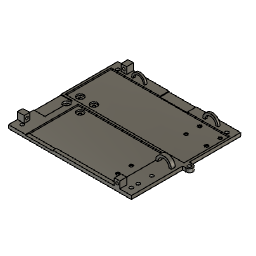
cocheV3 v2 (Autodesk Fusion 360 design; units mm, degrees)
Autodesk Fusion 360 part; units mm, degrees
sketch "Sketch1" plane through (0, 0, 0) normal (0, 0, 1) x (1, 0, 0)
  line L0 (-100, 120) -> (80, 120)
  line L1 (80, 120) -> (80, -40)
  line L2 (80, -40) -> (-100, -40)
  line L3 (-100, -40) -> (-100, 120)
  line L4 (80, 120) -> (80, 110)
  circle A0 centre (70, 110) radius 2
  circle A1 centre (70, -30) radius 2
  circle A2 centre (-90, 110) radius 2
  circle A3 centre (-90, -30) radius 2
  dimension "d1" = 180
  dimension "d2" = 160
  dimension "d3" = 4
  dimension "d4" = 4
  dimension "d5" = 4
  dimension "d6" = 4
  constraint horizontal L0
  constraint vertical L1
  constraint horizontal L2
  constraint vertical L3
  constraint coincident L1 L4.end
  measures "d1" distance of L0.start L0.end
  measures "d2" distance of L0.start L2.end
  measures "d3" diameter of A0
  measures "d4" diameter of A1
  measures "d5" diameter of A2
  measures "d6" diameter of A3
extrude "Extrude1" add sketch "Sketch1" along normal blind 5 contours L0 L1 L2 L3 L4 | A0 | A1 | A2 | A3
sketch "Sketch2" plane through (0, 0, 5) normal (0, 0, 1) x (-1, 0, 0)
  line L0 (-80, -120) -> (100, -120)
  line L1 (100, -120) -> (100, 40)
  line L2 (100, 40) -> (-80, 40)
  line L3 (-80, 40) -> (-80, -120)
  circle A0 centre (-70, -110) radius 2
  circle A1 centre (-70, 30) radius 2
  circle A2 centre (90, -110) radius 2
  circle A3 centre (90, 30) radius 2
  dimension "d9" = 4
  dimension "d10" = 4
  dimension "d11" = 4
  dimension "d12" = 4
  measures "d9" diameter of A0
  measures "d10" diameter of A1
  measures "d11" diameter of A2
  measures "d12" diameter of A3
extrude "Extrude2" add sketch "Sketch2" along normal blind 40 contours A0 | A1 | A2 | A3
sketch "Sketch3" plane through (0, 0, 5) normal (0, 0, 1) x (-1, 0, 0)
  circle A0 centre (90, 30) radius 2
  circle A1 centre (-70, 30) radius 2
  circle A2 centre (90, -110) radius 2
  circle A3 centre (-70, -110) radius 2
  line L0 (-80, -120) -> (100, -120)
  line L1 (100, -120) -> (100, 40)
  line L2 (100, 40) -> (-80, 40)
  line L3 (-80, 40) -> (-80, -120)
  line L4 (-77, -107) -> (97, -107)
  line L5 (97, -107) -> (97, -40)
  line L6 (97, -40) -> (-77, -40)
  line L7 (-77, -40) -> (-77, -107)
  line L8 (75, 35) -> (-53, 35)
  line L9 (-53, 35) -> (-53, -37)
  line L10 (-53, -37) -> (75, -37)
  line L11 (75, -37) -> (75, 35)
  dimension "d15" = 67
  dimension "d16" = 174
  dimension "d17" = 128
  dimension "d18" = 72
  constraint horizontal L4
  constraint vertical L5
  constraint horizontal L6
  constraint vertical L7
  constraint horizontal L8
  constraint vertical L9
  constraint horizontal L10
  constraint vertical L11
  measures "d15" distance of L4.start L6.end
  measures "d16" distance of L4.start L4.end
  measures "d17" distance of L8.start L8.end
  measures "d18" distance of L8.start L10.end
extrude "Extrude3" cut sketch "Sketch3" against normal blind 2 contours L4 L5 L6 L7 | L8 L9 L10 L11
sketch "Sketch4" plane through (0, 0, 5) normal (0, 0, 1) x (-1, 0, 0)
  line L0 (97, -107) -> (-77, -107)
  line L1 (-77, -107) -> (-77, -40)
  line L2 (-77, -40) -> (97, -40)
  line L3 (97, -40) -> (97, -107)
  line L4 (-53, 35) -> (75, 35)
  line L5 (75, 35) -> (75, -37)
  line L6 (75, -37) -> (-53, -37)
  line L7 (-53, -37) -> (-53, 35)
  circle A0 centre (90, 30) radius 2
  circle A1 centre (-70, 30) radius 2
  circle A2 centre (90, -110) radius 2
  circle A3 centre (-70, -110) radius 2
  line L8 (-80, -120) -> (100, -120)
  line L9 (100, -120) -> (100, 40)
  line L10 (100, 40) -> (-80, 40)
  line L11 (-80, 40) -> (-80, -120)
  line L12 (-80, -120) -> (-80, -70)
  line L13 (-80, -70) -> (-77, -70)
  circle A4 centre (-70, -80) radius 1.5
  circle A5 centre (-40, -80) radius 1.5
  circle A6 centre (-70, -100) radius 1.5
  circle A7 centre (-40, -100) radius 1.5
  circle A8 centre (-40, 20) radius 1.5
  circle A9 centre (-40, 0) radius 1.5
  circle A10 centre (-70, 20) radius 1.5
  circle A11 centre (-70, 0) radius 1.5
  point P0 (-40, 0)
  point P1 (-40, 20)
  point P2 (-70, 0)
  point P3 (-70, 20)
  dimension "d21" = 50
  dimension "d23" = 3
  dimension "d24" = 3
  dimension "d25" = 3
  dimension "d26" = 3
  dimension "d27" = 3
  dimension "d28" = 3
  dimension "d29" = 3
  dimension "d30" = 3
  constraint coincident L8.start L11.end
  constraint coincident L11 L12.end
  constraint perpendicular L1 L13
  constraint coincident L1 L13.end
  constraint symmetric L2 A4.centre P2
  constraint symmetric L2 A5.centre P0
  constraint symmetric L2 A6.centre P3
  constraint symmetric L2 A7.centre P1
  constraint coincident P1 A8.centre
  constraint coincident P0 A9.centre
  constraint coincident P3 A10.centre
  constraint coincident P2 A11.centre
  measures "d21" distance of L8.start L12.end
  measures "d23" diameter of A4
  measures "d24" diameter of A5
  measures "d25" diameter of A6
  measures "d26" diameter of A7
  measures "d27" diameter of A8
  measures "d28" diameter of A9
  measures "d29" diameter of A10
  measures "d30" diameter of A11
extrude "Extrude4" cut sketch "Sketch4" against normal blind 5 contours A4 | A5 | A6 | A7 | A8 | A9 | A10 | A11
sketch "Sketch5" plane through (0, 0, 5) normal (0, 0, 1) x (-1, 0, 0)
  circle A0 centre (-70, 20) radius 1.5
  circle A1 centre (-70, 0) radius 1.5
  line L0 (97, -107) -> (-77, -107)
  line L1 (-77, -107) -> (-77, -40)
  line L2 (-77, -40) -> (97, -40)
  line L3 (97, -40) -> (97, -107)
  line L4 (-53, 35) -> (75, 35)
  line L5 (75, 35) -> (75, -37)
  line L6 (75, -37) -> (-53, -37)
  line L7 (-53, -37) -> (-53, 35)
  circle A2 centre (90, 30) radius 2
  circle A3 centre (-70, 30) radius 2
  circle A4 centre (90, -110) radius 2
  circle A5 centre (-70, -110) radius 2
  line L8 (-80, -120) -> (100, -120)
  line L9 (100, -120) -> (100, 40)
  line L10 (100, 40) -> (-80, 40)
  line L11 (-80, 40) -> (-80, -120)
  circle A6 centre (-40, -100) radius 2.5
  circle A7 centre (-70, -100) radius 2.5
  circle A8 centre (-40, -80) radius 2.5
  circle A9 centre (-70, -80) radius 2.5
  circle A10 centre (-40, 0) radius 2.5
  circle A11 centre (-70, 0) radius 2.5
  circle A12 centre (-40, 20) radius 2.5
  circle A13 centre (-70, 20) radius 2.5
  dimension "d33" = 5
  dimension "d34" = 5
  dimension "d35" = 5
  dimension "d36" = 5
  dimension "d37" = 5
  dimension "d38" = 5
  dimension "d39" = 5
  dimension "d40" = 5
  constraint concentric A1 A11
  constraint concentric A0 A13
  measures "d33" diameter of A6
  measures "d34" diameter of A7
  measures "d35" diameter of A8
  measures "d36" diameter of A9
  measures "d37" diameter of A10
  measures "d38" diameter of A11
  measures "d39" diameter of A12
  measures "d40" diameter of A13
extrude "Extrude5" cut sketch "Sketch5" against normal blind 3 contours A6 | A7 | A8 | A9 | A10 | A11 | A12 | A13
sketch "Sketch6" plane through (0, 0, 0) normal (0, 0, 1) x (1, 0, 0)
sketch "Sketch7" plane through (0, 0, 5) normal (0, 0, 1) x (-1, 0, 0)
  circle A0 centre (-70, 20) radius 2.5
  circle A1 centre (-70, 0) radius 2.5
  line L0 (97, -107) -> (-77, -107)
  line L1 (-77, -107) -> (-77, -40)
  line L2 (-77, -40) -> (97, -40)
  line L3 (97, -40) -> (97, -107)
  line L4 (-53, 35) -> (75, 35)
  line L5 (75, 35) -> (75, -37)
  line L6 (75, -37) -> (-53, -37)
  line L7 (-53, -37) -> (-53, 35)
  circle A2 centre (90, 30) radius 2
  circle A3 centre (-70, 30) radius 2
  circle A4 centre (90, -110) radius 2
  circle A5 centre (-70, -110) radius 2
  line L8 (-80, -120) -> (100, -120)
  line L9 (100, -120) -> (100, 40)
  line L10 (100, 40) -> (-80, 40)
  line L11 (-80, 40) -> (-80, -120)
  line L12 (89.9439, -55) -> (59.9439, -25) construction
  line L13 (59.9439, -55) -> (89.9439, -25) construction
  circle A6 centre (85, -50) radius 2
  circle A7 centre (85, -30) radius 2
  circle A8 centre (65, -30) radius 2
  circle A9 centre (65, -50) radius 2
  point P0 (74.9439, -40)
  dimension "d43" = 30
  dimension "d44" = 30
  dimension "d45" = 4
  dimension "d46" = 4
  constraint coincident L12 P0
  constraint coincident L13 P0
  constraint coincident L2 P0
  constraint symmetric L5 A6 A9
  constraint symmetric L5 A7 A8
  measures "d43" distance of L13.start L12.end
  measures "d44" distance of L12.end L13.end
  measures "d45" diameter of A6
  measures "d46" diameter of A7
extrude "Extrude6" cut sketch "Sketch7" against normal blind 5 contours A6 | A7 | A8 | A9
sketch "Sketch8" plane through (0, 0, 5) normal (0, 0, 1) x (-1, 0, 0)
  circle A0 centre (85, -30) radius 2
  circle A1 centre (-70, 20) radius 2.5
  circle A2 centre (-70, 0) radius 2.5
  line L0 (97, -107) -> (-77, -107)
  line L1 (-77, -107) -> (-77, -40)
  line L2 (-77, -40) -> (97, -40)
  line L3 (97, -40) -> (97, -107)
  line L4 (-53, 35) -> (75, 35)
  line L5 (75, 35) -> (75, -37)
  line L6 (75, -37) -> (-53, -37)
  line L7 (-53, -37) -> (-53, 35)
  circle A3 centre (90, 30) radius 2
  circle A4 centre (-70, 30) radius 2
  circle A5 centre (90, -110) radius 2
  circle A6 centre (-70, -110) radius 2
  line L8 (-80, -120) -> (100, -120)
  line L9 (100, -120) -> (100, 40)
  line L10 (100, 40) -> (-80, 40)
  line L11 (-80, 40) -> (-80, -120)
  circle A7 centre (85, -30) radius 5
  circle A8 centre (85, -50) radius 5
  circle A9 centre (65, -30) radius 5
  circle A10 centre (65, -50) radius 5
  dimension "d49" = 10
  dimension "d50" = 10
  constraint concentric A0 A7
  constraint symmetric L5 A7 A9
  constraint symmetric L5 A8 A10
  measures "d49" diameter of A7
  measures "d50" diameter of A8
extrude "Extrude7" cut sketch "Sketch8" against normal blind 4 contours A7 | A8 | A9 | A10
sketch "Sketch9" plane through (0, 0, 5) normal (0, 0, 1) x (-1, 0, 0)
  circle A0 centre (85, -30) radius 5
  circle A1 centre (-70, 20) radius 2.5
  circle A2 centre (-70, 0) radius 2.5
  line L0 (97, -107) -> (-77, -107)
  line L1 (-77, -107) -> (-77, -40)
  line L2 (-77, -40) -> (97, -40)
  line L3 (97, -40) -> (97, -107)
  line L4 (-53, 35) -> (75, 35)
  line L5 (75, 35) -> (75, -37)
  line L6 (75, -37) -> (-53, -37)
  line L7 (-53, -37) -> (-53, 35)
  circle A3 centre (90, 30) radius 2
  circle A4 centre (-70, 30) radius 2
  circle A5 centre (90, -110) radius 2
  circle A6 centre (-70, -110) radius 2
  line L8 (-80, -120) -> (100, -120)
  line L9 (100, -120) -> (100, 40)
  line L10 (100, 40) -> (-80, 40)
  line L11 (-80, 40) -> (-80, -120)
  line L12 (44.2567, -115.3087) -> (40, -115.3087)
  line L13 (40, -115.3087) -> (40, -110)
  line L14 (40, -110) -> (44.2567, -110)
  line L15 (44.2567, -110) -> (44.2567, -115.3087)
  line L16 (-53, -28.3408) -> (-56.2998, -28.3408)
  line L17 (-56.2998, -28.3408) -> (-56.2998, -22.5656)
  line L18 (-56.2998, -22.5656) -> (-53, -22.5656)
  line L19 (-53, -22.5656) -> (-53, -28.3408)
  line L20 (-56.2998, -113.6101) -> (-53, -113.6101)
  line L21 (-53, -113.6101) -> (-53, -110.5526)
  line L22 (-53, -110.5526) -> (-56.2998, -110.5526)
  line L23 (-56.2998, -110.5526) -> (-56.2998, -113.6101)
  line L24 (-45.0891, -120) -> (-45.0891, -107)
  line L25 (-64.4531, -40) -> (-64.4531, 40)
  line L26 (30, -120) -> (30, -107)
  constraint horizontal L12
  constraint vertical L13
  constraint horizontal L14
  constraint vertical L15
  constraint horizontal L16
  constraint vertical L17
  constraint horizontal L18
  constraint vertical L19
  constraint coincident L7 L16.start
  constraint horizontal L20
  constraint vertical L21
  constraint horizontal L22
  constraint vertical L23
  constraint coincident L8 L24.start
  constraint coincident L0 L24.end
  constraint perpendicular L0 L24
  constraint coincident L2 L25.start
  constraint coincident L10 L25.end
  constraint perpendicular L10 L25
  constraint coincident L8 L26.start
  constraint coincident L0 L26.end
  constraint perpendicular L0 L26
revolve "Revolve1" add sketch "Sketch9" angle 180 about axis through (45.0891, 120, 5) along (0, -1, 0) contours L20 L21 L22 L23
sketch "Sketch10" plane through (0, 0, 5) normal (0, 0, 1) x (-1, 0, 0)
  line L0 (-56.2998, -110.5526) -> (-53, -110.5526)
  line L1 (-53, -110.5526) -> (-53, -113.6101)
  line L2 (-53, -113.6101) -> (-56.2998, -113.6101)
  line L3 (-56.2998, -113.6101) -> (-56.2998, -110.5526)
  line L4 (-37.1783, -110.5526) -> (-33.8784, -110.5526)
  line L5 (-33.8784, -110.5526) -> (-33.8784, -113.6101)
  line L6 (-33.8784, -113.6101) -> (-37.1783, -113.6101)
  line L7 (-37.1783, -113.6101) -> (-37.1783, -110.5526)
  circle A0 centre (85, -30) radius 5
  circle A1 centre (-70, 20) radius 2.5
  circle A2 centre (-70, 0) radius 2.5
  line L8 (97, -107) -> (-77, -107)
  line L9 (-77, -107) -> (-77, -40)
  line L10 (-77, -40) -> (97, -40)
  line L11 (97, -40) -> (97, -107)
  line L12 (-53, 35) -> (75, 35)
  line L13 (75, 35) -> (75, -37)
  line L14 (75, -37) -> (-53, -37)
  line L15 (-53, -37) -> (-53, 35)
  circle A3 centre (90, 30) radius 2
  circle A4 centre (-70, 30) radius 2
  circle A5 centre (90, -110) radius 2
  circle A6 centre (-70, -110) radius 2
  line L16 (-80, -120) -> (100, -120)
  line L17 (100, -120) -> (100, 40)
  line L18 (100, 40) -> (-80, 40)
  line L19 (-80, 40) -> (-80, -120)
  line L20 (70, -110) -> (67.5923, -110)
  line L21 (67.5923, -110) -> (67.5923, -113.0196)
  line L22 (67.5923, -113.0196) -> (70, -113.0196)
  line L23 (70, -113.0196) -> (70, -110)
  line L24 (60, -120) -> (60, -107)
  constraint horizontal L20
  constraint vertical L21
  constraint horizontal L22
  constraint vertical L23
  constraint coincident L16 L24.start
  constraint coincident L8 L24.end
  constraint perpendicular L8 L24
revolve "Revolve2" add sketch "Sketch10" angle 180 about axis through (-60, 120, 5) along (0, 1, 0) contours L20 L21 L22 L23
revolve "Revolve3" add sketch "Sketch9" angle 180 about axis through (64.4531, 40, 5) along (0, 1, 0) contours L7 L16 L17 L18 L19
sketch "Sketch11" plane through (80, 0, 0) normal (1, 0, 0) x (0, 1, 0)
  line L0 (-40, 0) -> (120, 0)
  line L1 (120, 0) -> (120, 5)
  line L2 (120, 5) -> (-40, 5)
  line L3 (-40, 5) -> (-40, 0)
  line L4 (35, 5) -> (45, 5)
  line L5 (45, 5) -> (45, 0)
  line L6 (45, 0) -> (35, 0)
  line L7 (35, 0) -> (35, 5)
  constraint horizontal L4
  constraint vertical L5
  constraint horizontal L6
  constraint vertical L7
  constraint coincident L0 L5.end
  constraint coincident L2 L4.start
extrude "Extrude8" add sketch "Sketch11" along normal blind 10 contours L0 L2 L4 L5 L6 L7
fillet "Fillet1" radius 5 1 edges at (90, 35, 2.5)
fillet "Fillet2" radius 5 1 edges at (90, 45, 2.5)
sketch "Sketch12" plane through (0, 0, 5) normal (0, 0, 1) x (-1, 0, 0)
  arc A0 (-85, -35) -> (-85, -45) centre (-85, -40) ccw
  line L0 (-85, -45) -> (-80, -45)
  line L1 (-80, -45) -> (-80, -120)
  line L2 (-80, -120) -> (100, -120)
  line L3 (100, -120) -> (100, 40)
  line L4 (100, 40) -> (-80, 40)
  line L5 (-80, 40) -> (-80, -35)
  line L6 (-80, -35) -> (-85, -35)
  line L7 (-75.9061, -28.3408) -> (-75.9061, -22.5656)
  line L8 (-75.9061, -22.5656) -> (-72.6063, -22.5656)
  line L9 (-72.6063, -22.5656) -> (-72.6063, -28.3408)
  line L10 (-72.6063, -28.3408) -> (-75.9061, -28.3408)
  line L11 (70, -113.0196) -> (67.5923, -113.0196)
  line L12 (67.5923, -113.0196) -> (67.5923, -110)
  line L13 (67.5923, -110) -> (70, -110)
  line L14 (70, -110) -> (70, -113.0196)
  line L15 (52.4077, -113.0196) -> (50, -113.0196)
  line L16 (50, -113.0196) -> (50, -110)
  line L17 (50, -110) -> (52.4077, -110)
  line L18 (52.4077, -110) -> (52.4077, -113.0196)
  line L19 (-56.2998, -110.5526) -> (-53, -110.5526)
  line L20 (-53, -110.5526) -> (-53, -113.6101)
  line L21 (-53, -113.6101) -> (-56.2998, -113.6101)
  line L22 (-56.2998, -113.6101) -> (-56.2998, -110.5526)
  line L23 (-37.1783, -110.5526) -> (-33.8784, -110.5526)
  line L24 (-33.8784, -110.5526) -> (-33.8784, -113.6101)
  line L25 (-33.8784, -113.6101) -> (-37.1783, -113.6101)
  line L26 (-37.1783, -113.6101) -> (-37.1783, -110.5526)
  circle A1 centre (85, -30) radius 5
  circle A2 centre (-70, 20) radius 2.5
  circle A3 centre (-70, 0) radius 2.5
  line L27 (97, -107) -> (-77, -107)
  line L28 (-77, -107) -> (-77, -40)
  line L29 (-77, -40) -> (97, -40)
  line L30 (97, -40) -> (97, -107)
  line L31 (-53, -28.3408) -> (-56.2998, -28.3408)
  line L32 (-56.2998, -28.3408) -> (-56.2998, -22.5656)
  line L33 (-56.2998, -22.5656) -> (-53, -22.5656)
  line L34 (-53, -22.5656) -> (-53, 35)
  line L35 (-53, 35) -> (75, 35)
  line L36 (75, 35) -> (75, -37)
  line L37 (75, -37) -> (-53, -37)
  line L38 (-53, -37) -> (-53, -28.3408)
  circle A4 centre (90, 30) radius 2
  circle A5 centre (-70, 30) radius 2
  circle A6 centre (90, -110) radius 2
  circle A7 centre (-70, -110) radius 2
  circle A8 centre (-85, -40) radius 2.589
  constraint concentric A0 A8
hole "Hole1" at (85, 40, 5) direction (0, 0, -1) diameter 5 depth 11 tip angle 118
extrude "Extrude9" cut 1 faces at (70.9758, -29.5466, 45) along direction (0, 0, -1) blind 41
extrude "Extrude10" add sketch "Sketch9" against normal blind 1 contours A4
extrude "Extrude11" cut 3 faces at (-90.4157, 109.2801, 45) (-89.0242, -29.5466, 45) (69.5843, 109.2801, 45) along direction (0, 0, -1) blind 40
sketch "Sketch13" plane through (0, 0, 5) normal (0, 0, 1) x (-1, 0, 0)
  circle A0 centre (-70, 30) radius 2.5
  circle A1 centre (90, 30) radius 2.5
  circle A2 centre (-70, -110) radius 2.5
  circle A3 centre (90, -110) radius 2.5
  dimension "d69" = 5
  dimension "d70" = 5
  dimension "d71" = 5
  dimension "d72" = 5
  measures "d69" diameter of A0
  measures "d70" diameter of A1
  measures "d71" diameter of A2
  measures "d72" diameter of A3
extrude "Extrude12" cut sketch "Sketch13" against normal blind 3
sketch "Sketch14" plane through (0, 0, 5) normal (0, 0, 1) x (-1, 0, 0)
  line L0 (100, -37) -> (83.6937, -37)
  line L1 (83.6937, -37) -> (83.6937, 3)
  line L2 (83.6937, 3) -> (100, 3)
  line L3 (100, 3) -> (100, -37)
  line L4 (86, 40) -> (45.9685, 40)
  line L5 (45.9685, 40) -> (45.9685, 23.7)
  line L6 (45.9685, 23.7) -> (86, 23.7)
  line L7 (86, 23.7) -> (86, 40)
  line L8 (25, -120) -> (-15, -120)
  line L9 (-15, -120) -> (-15, -105)
  line L10 (-15, -105) -> (25, -105)
  line L11 (25, -105) -> (25, -120)
  dimension "d75" = 40
  dimension "d76" = 16.3
  constraint horizontal L0
  constraint vertical L1
  constraint horizontal L2
  constraint vertical L3
  constraint horizontal L4
  constraint vertical L5
  constraint horizontal L6
  constraint vertical L7
  constraint horizontal L8
  constraint vertical L9
  constraint horizontal L10
  constraint vertical L11
  measures "d75" distance of L0.start L2.end
  measures "d76" distance of L4.start L6.end
extrude "Extrude13" cut sketch "Sketch14" against normal blind 1
extrude "Extrude14" add sketch "Sketch14" against normal blind 1 contours L4 L5 L6 L7
sketch "Sketch15" plane through (0, 0, 5) normal (0, 0, 1) x (-1, 0, 0)
  line L0 (35, 40) -> (75, 40)
  line L1 (75, 40) -> (75, 23)
  line L2 (75, 23) -> (35, 23)
  line L3 (35, 23) -> (35, 40)
  constraint horizontal L0
  constraint vertical L1
  constraint horizontal L2
  constraint vertical L3
extrude "Extrude15" cut sketch "Sketch15" against normal blind 1
sketch "Sketch16" plane through (0, 0, 5) normal (0, 0, 1) x (-1, 0, 0)
  line L0 (-55, 40) -> (-63, 40)
  line L1 (-63, 40) -> (-63, 30)
  line L2 (-63, 30) -> (-55, 30)
  line L3 (-55, 30) -> (-55, 40)
  line L4 (100, 27) -> (90, 27)
  line L5 (90, 27) -> (90, 19)
  line L6 (90, 19) -> (100, 19)
  line L7 (100, 19) -> (100, 27)
  line L8 (85, -120) -> (77, -120)
  line L9 (77, -120) -> (77, -110)
  line L10 (77, -110) -> (85, -110)
  line L11 (85, -110) -> (85, -120)
  constraint horizontal L0
  constraint vertical L1
  constraint horizontal L2
  constraint vertical L3
  constraint horizontal L4
  constraint vertical L5
  constraint horizontal L6
  constraint vertical L7
  constraint horizontal L8
  constraint vertical L9
  constraint horizontal L10
  constraint vertical L11
extrude "Extrude16" add sketch "Sketch16" along normal blind 10
sketch "Sketch17" plane through (0, -40, 0) normal (0, -1, 0) x (1, 0, 0)
  line L0 (-35, 5) -> (-35, 4)
  line L1 (-35, 4) -> (-75, 4)
  line L2 (-75, 4) -> (-75, 5)
  line L3 (-75, 5) -> (-100, 5)
  line L4 (-100, 5) -> (-100, 0)
  line L5 (-100, 0) -> (80, 0)
  line L6 (80, 0) -> (80, 5)
  line L7 (80, 5) -> (63, 5)
  line L8 (63, 5) -> (63, 15)
  line L9 (63, 15) -> (55, 15)
  line L10 (55, 15) -> (55, 5)
  line L11 (55, 5) -> (-35, 5)
  circle A0 centre (59.0319, 10) radius 1.975
  dimension "d85" = 3.95
  measures "d85" diameter of A0
extrude "Extrude17" cut sketch "Sketch17" against normal blind 17 contours A0
sketch "Sketch18" plane through (-90, 0, 0) normal (1, 0, 0) x (0, 1, 0)
  line L0 (-27, 5) -> (-19, 5)
  line L1 (-19, 5) -> (-19, 15)
  line L2 (-19, 15) -> (-27, 15)
  line L3 (-27, 15) -> (-27, 5)
  circle A0 centre (-23, 10) radius 1.975
  dimension "d88" = 3.95
  measures "d88" diameter of A0
extrude "Extrude18" cut sketch "Sketch18" against normal blind 26 contours A0
sketch "Sketch19" plane through (0, 120, 0) normal (0, 1, 0) x (-1, 0, 0)
  line L0 (25, 5) -> (25, 4)
  line L1 (25, 4) -> (-15, 4)
  line L2 (-15, 4) -> (-15, 5)
  line L3 (-15, 5) -> (-80, 5)
  line L4 (-80, 5) -> (-80, 0)
  line L5 (-80, 0) -> (100, 0)
  line L6 (100, 0) -> (100, 5)
  line L7 (100, 5) -> (85, 5)
  line L8 (85, 5) -> (85, 15)
  line L9 (85, 15) -> (77, 15)
  line L10 (77, 15) -> (77, 5)
  line L11 (77, 5) -> (25, 5)
  circle A0 centre (81, 10) radius 1.975
  dimension "d91" = 3.95
  measures "d91" diameter of A0
extrude "Extrude19" cut sketch "Sketch19" against normal blind 12 contours A0
